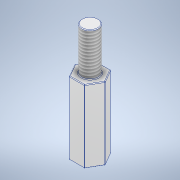
# Autodesk Inventor part: 11mm_standoff
Saved by Autodesk Inventor 2020.2 (Build 242310000, 310)
## iProperties
Created: 2020-04-11
Part Number: 11mm_standoff
Material: Aluminum 6061
Document SubType Name: Modeling
Designer: agmlego
Mass: 0.44154 g
Surface Area: 2.6944 cm^2
Volume: 0.163533 cm^3
Density: 2.7 g/cm^3
Appearance: Aluminum - Flat
Author: agmlego
Autodesk Inventor part; units mm, degrees
ref_plane "YZ Plane" through (0, 0, 0) normal (1, 0, 0) x (0, 1, 0)
ref_plane "XZ Plane" through (0, 0, 0) normal (0, 1, 0) x (-1, 0, 0)
ref_plane "XY Plane" through (0, 0, 0) normal (0, 0, 1) x (1, 0, 0)
sketch "Sketch1" plane through (0, 0, 0) normal (0, 1, 0) x (-1, 0, 0)
  line L0 (2.3094, 0) -> (1.1547, -2)
  line L1 (1.1547, -2) -> (-1.1547, -2)
  line L2 (-1.1547, -2) -> (-2.3094, 0)
  line L3 (-2.3094, 0) -> (-1.1547, 2)
  line L4 (-1.1547, 2) -> (1.1547, 2)
  line L5 (1.1547, 2) -> (2.3094, 0)
  point P0 (0, 0)
  point P1 (0, 0)
  dimension "d0" = 4
  constraints: 12 end point, 1 coincident, 1 horizontal, 13 other
  measures "d0" distance between parallel lines of L1 L4
extrude "Extrusion1" add sketch "Sketch1" along normal blind 11
sketch "Sketch2" plane through (0, 11, 0) normal (0, 1, 0) x (1, 0, 0)
  circle A0 centre (0, 0) radius 1.25
  dimension "d3" = 2.5
  constraints: 1 centre point, 1 coincident
  measures "d3" diameter of A0
extrude "Extrusion2" add sketch "Sketch2" along normal blind 6.5
thread "Thread1" size "M2.5x0.45" class "6g" standard "ANSI Metric M Profile" full length
sketch "Sketch3" plane through (0, 0, 0) normal (0, -1, 0) x (1, 0, 0)
  point P0 (0, 0)
  point P1 (0, 0)
  constraints: 1 coincident
hole "Hole1" at (0, 0, 0) direction (0, 1, 0) diameter 2.013 depth 6.5 start extended yes thread size "M2.5x0.45" class "6H" standard "ANSI Metric M Profile"
fillet "Fillet1" radius 0.1 21 edges at (-1.1547, 5.5, 2) (-2.3094, 5.5, 0) (-1.1547, 5.5, -2) (1.1547, 5.5, -2) (2.3094, 5.5, 0) (1.1547, 5.5, 2) (0, 0, 2) (1.7321, 0, 1) (1.7321, 0, -1) (0, 0, -2) (-1.7321, 0, -1) (-1.7321, 0, 1) (0, 0, 1.0065) (1.7321, 11, 1) (0, 11, 2) (-1.7321, 11, 1) (-1.7321, 11, -1) (0, 11, -2) (1.7321, 11, -1) (-1.25, 17.5, 0) (-1.25, 11, 0)
body "Solid1"
